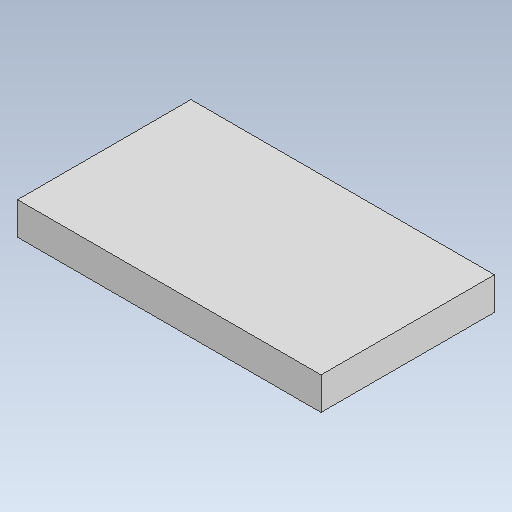
# Autodesk Inventor part: woodForkFrontSupport
Saved by Autodesk Inventor 2021 (Build 250183000, 183)
## iProperties
Created: 2020-07-02
Part Number: woodForkFrontSupport
Material: Generic
Document SubType Name: Modeling
Designer: robst
Density: 1 g/cm^3
Appearance: Default
Author: robst
Autodesk Inventor part; units mm, degrees
ref_plane "YZ Plane" through (0, 0, 0) normal (1, 0, 0) x (0, 1, 0)
ref_plane "XZ Plane" through (0, 0, 0) normal (0, 1, 0) x (-1, 0, 0)
ref_plane "Work Plane1" through (0, 0, 0) normal (0, 0, 1) x (1, 0, 0)
sketch "Sketch1" plane through (0, 0, 0) normal (0, 0, 1) x (1, 0, 0)
  line L0 (82.55, 101.6) -> (82.55, -101.6) projected
  line L1 (101.6, 101.6) -> (-101.6, 101.6) projected
  line L2 (-95.25, 101.6) -> (-95.25, -101.6) projected
  line L3 (82.55, 101.6) -> (-95.25, 101.6)
  line L4 (-95.25, 101.6) -> (-95.25, 82.55)
  line L5 (-95.25, 82.55) -> (82.55, 82.55)
  line L6 (82.55, 82.55) -> (82.55, 101.6)
  point P0 (0, 0)
  point P1 (82.55, 82.55)
  dimension "d0" = 19.05
  constraints: 8 end point, 2 parallel, 1 horizontal, 1 perpendicular, 1 point on line
  measures "d0" distance between parallel lines of L5 L1
extrude "Extrusion1" add sketch "Sketch1" along normal blind 101.6
body "Solid1"
